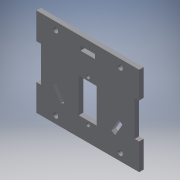
# Autodesk Inventor part: Camera pan base
Saved by Autodesk Inventor 2018 (Build 220112000, 112)
## iProperties
Created: 2018-06-25
Part Number: Camera pan base
Material: Generic
Document SubType Name: Modeling
Designer: Ajith Thomas
Density: 1 g/cm^3
Appearance: Default
Author: Ajith Thomas
Autodesk Inventor part; units mm, degrees
ref_plane "YZ Plane" through (0, 0, 0) normal (1, 0, 0) x (0, 1, 0)
ref_plane "XZ Plane" through (0, 0, 0) normal (0, 1, 0) x (-1, 0, 0)
ref_plane "XY Plane" through (0, 0, 0) normal (0, 0, 1) x (1, 0, 0)
sketch "Sketch1" plane through (0, 0, 0) normal (0, 0, 1) x (1, 0, 0)
  arc A0 (8.3864, -11.505) -> (3.6136, -11.505) centre (6, -6) ccw construction
  line L0 (-28.75, -36) -> (40.75, -36)
  line L1 (40.75, -36) -> (40.75, 24)
  line L2 (40.75, 24) -> (-28.75, 24)
  line L3 (-28.75, 24) -> (-28.75, -36)
  line L4 (-28.75, -36) -> (40.75, 24) construction
  line L5 (40.75, -36) -> (-28.75, 24) construction
  line L6 (12, 0) -> (0, 0) projected
  line L7 (0, 0) -> (0, -23) projected
  line L8 (0, -23) -> (12, -23) projected
  line L9 (12, -23) -> (12, 0) projected
  line L10 (-0.1, -23.1) -> (12.1, -23.1)
  line L11 (12.1, -23.1) -> (12.1, 0.1)
  line L12 (12.1, 0.1) -> (-0.1, 0.1)
  line L13 (-0.1, 0.1) -> (-0.1, -23.1)
  line L14 (-28.75, -6) -> (40.75, -6) construction
  line L15 (6, -36) -> (6, 24) construction
  line L16 (-28.75, -18) -> (-25.75, -18)
  line L17 (-25.75, -18) -> (-25.75, 6)
  line L18 (-25.75, 6) -> (-28.75, 6)
  line L19 (-28.75, 6) -> (-28.75, -18)
  line L20 (40.75, -18) -> (37.75, -18)
  line L21 (37.75, -18) -> (37.75, 6)
  line L22 (37.75, 6) -> (40.75, 6)
  line L23 (40.75, 6) -> (40.75, -18)
  arc A1 (6.5, -26.804) -> (5.5, -26.804) centre (6, -25.55) ccw construction
  arc A2 (5.5, 3.804) -> (6.5, 3.804) centre (6, 2.55) ccw construction
  circle A3 centre (6, -25.55) radius 1.35
  circle A4 centre (6, 2.55) radius 1.35
  dimension "d0" = 69.5
  dimension "d1" = 60
  dimension "d2" = 0.1
  dimension "d3" = 0.1
  dimension "d4" = 0.1
  dimension "d5" = 0.1
  dimension "d6" = 12
  dimension "d7" = 12
  dimension "d8" = 3
  constraints: 40 end point, 6 midpoint, 6 parallel, 4 symmetric about line, 3 horizontal, 3 perpendicular, 2 centre point, 2 coincident, 2 concentric, 1 point on line
  measures "d0" distance of L2.end L1.end
  measures "d1" distance of L1.end L0.end
  measures "d2" distance between parallel lines of L10 L8
  measures "d3" distance between parallel lines of L7 L13
  measures "d4" distance between parallel lines of L6 L12
  measures "d5" distance between parallel lines of L9 L11
  measures "d6" distance between parallel lines of L16 L14
  measures "d7" distance between parallel lines of L18 L14
  measures "d8" distance between parallel lines of L3 L17
extrude "Extrusion1" add sketch "Sketch1" along normal blind 3 contours L3 L16 L17 L18 L2 L1 L22 L21 L20 L0
sketch "Sketch2" plane through (0, 0, 0) normal (0, 0, -1) x (-1, 0, 0)
  circle A0 centre (15.85, 19) radius 1.8 projected
  circle A1 centre (-27.85, 19) radius 1.8 projected
  circle A2 centre (-27.85, -31) radius 1.8 projected
  circle A3 centre (15.85, -31) radius 1.8 projected
  point P0 (0, 0)
extrude "Extrusion2" cut sketch "Sketch2" against normal blind 7.7625
sketch "Sketch3" plane through (0, 0, 3) normal (0, 0, 1) x (1, 0, 0)
  line L0 (-14.9463, -12.3199) -> (-9.9463, -20.9801) construction
  line L1 (-17.5444, -13.8199) -> (-12.5444, -22.4801) construction
  line L2 (-12.5444, -22.4801) -> (-9.9463, -20.9801) construction
  line L3 (-17.5444, -13.8199) -> (-14.9463, -12.3199) construction
  line L4 (29.5444, -13.8199) -> (26.9463, -12.3199) construction
  line L5 (24.5444, -22.4801) -> (21.9463, -20.9801) construction
  line L6 (21.9463, -20.9801) -> (26.9463, -12.3199) construction
  line L7 (24.5444, -22.4801) -> (29.5444, -13.8199) construction
  line L8 (11, 15.3) -> (1, 15.3) construction
  line L9 (11, 18.3) -> (1, 18.3) construction
  line L10 (11, 18.3) -> (11, 15.3) construction
  line L11 (1, 18.3) -> (1, 15.3) construction
  line L12 (26.9646, -12.3882) -> (29.4761, -13.8382)
  line L13 (29.4761, -13.8382) -> (24.5261, -22.4118)
  line L14 (24.5261, -22.4118) -> (22.0146, -20.9618)
  line L15 (22.0146, -20.9618) -> (26.9646, -12.3882)
  line L16 (-10.0146, -20.9618) -> (-14.9646, -12.3882)
  line L17 (-14.9646, -12.3882) -> (-17.4761, -13.8382)
  line L18 (-17.4761, -13.8382) -> (-12.5261, -22.4118)
  line L19 (-12.5261, -22.4118) -> (-10.0146, -20.9618)
  line L20 (1.05, 15.35) -> (10.95, 15.35)
  line L21 (10.95, 15.35) -> (10.95, 18.25)
  line L22 (10.95, 18.25) -> (1.05, 18.25)
  line L23 (1.05, 18.25) -> (1.05, 15.35)
  point P0 (0, 0)
  dimension "d13" = 0.05
  dimension "d14" = 0.05
  dimension "d15" = 0.05
  constraints: 24 end point, 9 other
  measures "d13" distance between parallel lines of L6 L15
  measures "d14" distance between parallel lines of L0 L16
  measures "d15" distance between parallel lines of L8 L20
extrude "Extrusion3" cut sketch "Sketch3" against normal blind 10
body "Solid1"
